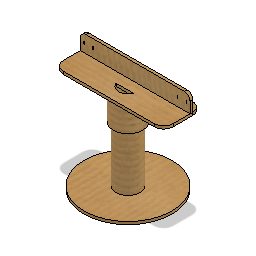
Beamforming_Antenna_Structure (Autodesk Fusion 360 design; units mm, degrees)
Autodesk Fusion 360 part; units mm, degrees
sketch "Sketch1" plane through (0, 0, 0) normal (0, 1, 0) x (1, 0, 0) in component "Base"
  circle A0 centre (0, 0) radius 79.0913
  dimension "d1" = 158.1826
  constraint coincident A0.centre origin
  measures "d1" diameter of A0
extrude "Extrude1" add sketch "Sketch1" along normal blind 5 makes body 1 in component "Base"
sketch "Sketch3" plane through (0, 0, 0) normal (0, 1, 0) x (1, 0, 0) in component "Mast"
  circle A0 centre (0, 0) radius 21.6265
  circle A1 centre (0, 0) radius 16.6265
  dimension "d6" = 43.2531
  dimension "d63" = 0
  dimension "d64" = 0
  dimension "d65" = 0
  constraint coincident A0.centre A1.centre
  measures "d6" diameter of A0
extrude "Extrude1'" add sketch "Sketch3" along normal blind 150 separate body makes body 2 in component "Mast"
sketch "Sketch1 (2)" plane through (0, 0, 0) normal (0, 1, 0) x (1, 0, 0) in component "Neck"
  circle A0 centre (0, 0) radius 21.6265
  circle A1 centre (0, 0) radius 26.6265
  dimension "d22" = 43.2531
  dimension "d23" = 5
  constraint coincident A0.centre A1.centre
  measures "d22" diameter of A0
extrude "Extrude1''" add sketch "Sketch1 (2)" against normal blind 50 separate body makes body 3 in component "Neck"
sketch "Sketch2" plane through (0, 0, 0) normal (0, 1, 0) x (1, 0, 0) in component "Beam"
  line L0 (-98.8641, 34.6024) -> (98.8641, 34.6024)
  line L1 (98.8641, 34.6024) -> (98.8641, -34.6024)
  line L2 (98.8641, -34.6024) -> (-98.8641, -34.6024)
  line L3 (-98.8641, -34.6024) -> (-98.8641, 34.6024)
  dimension "d29" = 197.7283
  dimension "d30" = 98.8641
  dimension "d31" = 69.2049
  dimension "d32" = 34.6024
  dimension "d59" = 0
  dimension "d60" = 0
  dimension "d61" = 0
  dimension "d101" = 0
  dimension "d102" = 0
  dimension "d103" = 0
  constraint horizontal L0
  constraint vertical L1
  constraint horizontal L2
  constraint vertical L3
  measures "d29" distance of L0.start L0.end
  measures "d30" distance of origin L3
  measures "d31" distance of L0 L2
  measures "d32" distance of origin L2
extrude "Extrude1'''" add sketch "Sketch2" along normal blind 5 separate body makes body 4 in component "Beam"
sketch "Sketch4" plane through (0, 5, 0) normal (0, 1, 0) x (-1, 0, 0) in component "Beam"
  line L0 (98.8641, 34.6024) -> (-98.8641, 34.6024)
  line L1 (-98.8641, 34.6024) -> (-98.8641, -34.6024)
  line L2 (-98.8641, -34.6024) -> (98.8641, -34.6024)
  line L3 (98.8641, -34.6024) -> (98.8641, 34.6024)
  circle A0 centre (0, 0) radius 26.6265
  circle A1 centre (0, 0) radius 26.6265
  circle A2 centre (0, 0) radius 21.6265
  circle A3 centre (0, 0) radius 26.6265
  circle A4 centre (0, 0) radius 16.6265
  line L4 (15.5771, 5.8133) -> (-15.5771, 5.8133)
  point P0 (0, 5.8133)
  point P1 (0, 16.6265)
  dimension "d80" = 10.8133
  constraint coincident A4 L4.start
  constraint coincident A4 L4.end
  constraint horizontal L4
  constraint midpoint L4 P0
  constraint coincident A4 P1
  constraint vertical P0 P1
  measures "d80" distance of P0 P1
extrude "Extrude2" cut sketch "Sketch4" against normal blind 9 contours A4 L4 picked at (-2.8933, 10.4159) bodies 4 in component "Beam"
fillet "Fillet1" radius 17.3012 4 edges at (98.8641, 2.5, 34.6024) (98.8641, 2.5, -34.6024) (-98.8641, 2.5, 34.6024) (-98.8641, 2.5, -34.6024) on bodies 4 in component "Beam"
sketch "Sketch2 (2)" plane through (0, 0, 0) normal (0, 0, 1) x (1, 0, 0) in component "Lip"
  line L0 (-98.8641, 0) -> (98.8641, 0)
  line L1 (98.8641, 0) -> (98.8641, 30)
  line L2 (98.8641, 30) -> (-98.8641, 30)
  line L3 (-98.8641, 30) -> (-98.8641, 0)
  dimension "d92" = 197.7283
  dimension "d93" = 30
  dimension "d94" = 98.8641
  dimension "d97" = 0
  dimension "d98" = 0
  dimension "d99" = 0
  constraint horizontal L0
  constraint vertical L1
  constraint horizontal L2
  constraint vertical L3
  measures "d92" distance of L0.start L0.end
  measures "d93" distance of L0.start L2.end
  measures "d94" distance of origin L3
extrude "Extrude2'" add sketch "Sketch2 (2)" against normal blind 5 separate body makes body 5 in component "Lip"
sketch "Sketch5" plane through (0, 5, 0) normal (0, 1, 0) x (-1, 0, 0) in component "Beam"
  line L0 (98.8641, -17.3012) -> (98.8641, 17.3012)
  line L1 (81.5629, 34.6024) -> (-81.5629, 34.6024)
  line L2 (-98.8641, 17.3012) -> (-98.8641, -17.3012)
  line L3 (-81.5629, -34.6024) -> (81.5629, -34.6024)
  line L4 (15.5771, 5.8133) -> (-15.5771, 5.8133)
  arc A0 (15.5771, 5.8133) -> (-15.5771, 5.8133) centre (0, 0) ccw
  arc A1 (81.5629, -34.6024) -> (98.8641, -17.3012) centre (81.5629, -17.3012) ccw
  arc A2 (98.8641, 17.3012) -> (81.5629, 34.6024) centre (81.5629, 17.3012) ccw
  arc A3 (-81.5629, 34.6024) -> (-98.8641, 17.3012) centre (-81.5629, 17.3012) ccw
  arc A4 (-98.8641, -17.3012) -> (-81.5629, -34.6024) centre (-81.5629, -17.3012) ccw
sketch "Sketch6" plane through (0, 5, 0) normal (0, 1, 0) x (-1, 0, 0) in component "Beam"
  line L0 (79.4745, 5) -> (79.4745, -6) construction
  point P0 (84.2114, -5)
  point P1 (74.7376, -5)
  point P2 (-93.6851, -5)
  dimension "d114" = 84.2114
  dimension "d118" = 168.4227
  dimension "d119" = 0
  constraint vertical L0
  constraint symmetric P0 L0 P1
  measures "d114" horizontal distance of origin P0
fillet "Fillet1'" radius 10 2 edges at (-98.8641, 30, -2.5) (98.8641, 30, -2.5) on bodies 5 in component "Lip"
sketch "Sketch3 (2)" plane through (0, 0, 0) normal (0, 0, 1) x (1, 0, 0) in component "Lip"
  line L0 (-98.8641, 20) -> (-98.8641, 0)
  line L1 (-98.8641, 0) -> (98.8641, 0)
  line L2 (98.8641, 0) -> (98.8641, 20)
  line L3 (88.8641, 30) -> (-88.8641, 30)
  line L4 (-98.8641, 0) -> (98.8641, 0)
  line L5 (-76.7114, 17) -> (-75.7114, 17)
  line L6 (-75.7114, 17) -> (-75.7114, 13)
  line L7 (-75.7114, 13) -> (-76.7114, 13)
  line L8 (-76.7114, 13) -> (-76.7114, 17)
  line L9 (-84.2114, 15) -> (-84.2114, 18) construction
  line L10 (-91.7114, 13) -> (-91.7114, 17)
  line L11 (-92.7114, 17) -> (-92.7114, 13)
  line L12 (-91.7114, 17) -> (-92.7114, 17)
  line L13 (-92.7114, 13) -> (-91.7114, 13)
  arc A0 (98.8641, 20) -> (88.8641, 30) centre (88.8641, 20) ccw
  arc A1 (-88.8641, 30) -> (-98.8641, 20) centre (-88.8641, 20) ccw
  point P0 (-84.2114, 15)
  dimension "d120" = 15
  dimension "d121" = 84.2114
  dimension "d122" = 4
  dimension "d123" = 1
  dimension "d124" = 2
  dimension "d125" = 7.5
  dimension "d126" = 3
  constraint horizontal L5
  constraint vertical L6
  constraint horizontal L7
  constraint vertical L8
  constraint vertical L9
  constraint coincident P0 L9.start
  constraint symmetric L5.start L9 L10.end
  constraint symmetric L5.end L9 L11.start
  constraint symmetric L6.end L9 L11.end
  constraint symmetric L7.end L9 L10.start
  measures "d120" distance of P0 L4
  measures "d121" horizontal distance of origin L9.start
  measures "d122" distance of L5.start L7.end
  measures "d123" distance of L5.start L5.end
  measures "d124" distance of P0 L5
  measures "d125" distance of P0 L8
  measures "d126" distance of P0 L9.end
extrude "Extrude3" cut sketch "Sketch3 (2)" against normal blind 13 contours L5 L6 L7 L8 | L10 L11 L12 L13 bodies 5 in component "Lip"
pattern_linear "R-Pattern1" count 1 spacing 168.4227 along (-1, 0, 0) of "Extrude3" in component "Lip"
pattern_linear "R-Pattern2" count 2 spacing 168.4227 along (1, 0, 0) of "Extrude3" in component "Lip"
component "Lower_Half" placed x (1, 0, 0) y (0, 1, 0) z (0, 0, 1) at (0, 0, 0)
component "Upper_Half" placed x (1, 0, 0) y (0, 1, 0) z (0, 0, 1) at (0, 0, 0)
component "Base" placed x (1, 0, 0) y (0, 1, 0) z (0, 0, 1) at (0, 0, 0) in component "Lower_Half"
component "Mast" placed x (1, 0, 0) y (0, 1, 0) z (0, 0, 1) at (0, 5, 0) in component "Lower_Half"
component "Neck" placed x (1, 0, 0) y (0, 1, 0) z (0, 0, 1) at (0, 155, 0) in component "Upper_Half"
component "Beam" placed x (1, 0, 0) y (0, 1, 0) z (0, 0, 1) at (0, 155, 0) in component "Upper_Half"
component "Lip" placed x (1, 0, 0) y (0, 1, 0) z (0, 0, 1) at (0, 160, -12.9759) in component "Upper_Half"
equation "d1 = base_diameter"
equation "d2 = width"
equation "d6 = mast_diameter"
equation "d7 = -width"
equation "mast_diameter = 0.625 * beam_width"
equation "base_diameter = 0.8 * beam_length"
equation "width = 5 mm"
equation "neck_height = mast_height / 3"
equation "d22 = mast_diameter"
equation "d23 = width"
equation "d24 = -neck_height"
equation "beam_width = 0.35 * ( antenna_elements - 1 ) ^ -0.7 * beam_length"
equation "beam_length = ( antenna_elements - 1 ) * array_distancing * 1.174"
equation "d29 = beam_length"
equation "d30 = beam_length / 2"
equation "d31 = beam_width"
equation "d32 = beam_width / 2"
equation "d33 = width"
equation "d80 = gap_size"
equation "gap_size = 0.25 * mast_diameter"
equation "d84 = beam_width / 4"
equation "lip_height = 30 mm"
equation "d92 = beam_length"
equation "d93 = lip_height"
equation "d94 = beam_length / 2"
equation "d95 = -width"
equation "d107 = 0.75 / 4 * beam_width"
equation "array_distancing = wavelength / 2"
equation "frequency = 890" comment "Frequency in MHz"
equation "lightspeed = 299792458"
equation "wavelength = ( lightspeed / frequency / 1E+06 ) * 1 m"
equation "d114 = array_distancing / 2"
equation "antenna_elements = 2"
equation "d116 = antenna_elements / 2"
equation "d118 = array_distancing"
equation "d120 = lip_height / 2"
equation "d121 = array_distancing / 2"
equation "d125 = 15 mm / 2"
equation "d129 = antenna_elements / 2"
equation "d131 = -array_distancing"
equation "d133 = antenna_elements / 2 + 1"
equation "d135 = array_distancing"
equation "mast_height = 150 mm"
